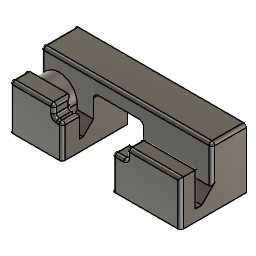
GBP - Cutting Tool v15 (Autodesk Fusion 360 design; units mm, degrees)
Autodesk Fusion 360 part; units mm, degrees
sketch "Boceto1" plane through (0, 0, 0) normal (0, 0, 1) x (1, 0, 0)
  line L0 (0, 7.25) -> (30, 7.25)
  line L1 (30, 7.25) -> (30, -4.25)
  line L2 (30, -4.25) -> (0, -4.25)
  line L3 (0, -4.25) -> (0, 7.25)
  dimension "d1" = 30
  dimension "d2" = 11.5
  dimension "d3" = 7.25
  constraint horizontal L0
  constraint vertical L1
  constraint horizontal L2
  constraint vertical L3
  measures "d1" distance of L0.start L0.end
  measures "d2" distance of L0.end L1.end
  measures "d3" distance of origin L0.start
extrude "Extruir1" add sketch "Boceto1" along normal blind 2
sketch "Boceto2" plane through (0, 0, 2) normal (0, 0, 1) x (-1, 0, 0)
  line L0 (0, 4.25) -> (-30, 4.25)
  line L1 (-30, 4.25) -> (-30, -7.25)
  line L2 (-30, -7.25) -> (0, -7.25)
  line L3 (0, -7.25) -> (0, 4.25)
  line L4 (0, -1.23) -> (-30, -1.23)
  line L5 (0, 1.23) -> (-30, 1.23)
  line L6 (-6.35, -1.23) -> (-6.35, 1.23)
  line L7 (-9.2, -1.23) -> (-9.2, 1.23)
  line L8 (-18, -1.23) -> (-18, 1.23)
  line L9 (0, -0.5) -> (-30, -0.5)
  dimension "d6" = 2.46
  dimension "d7" = 1.23
  dimension "d8" = 6.35
  dimension "d9" = 9.2
  dimension "d10" = 18
  constraint coincident L3 L4.start
  constraint coincident L1 L4.end
  constraint perpendicular L1 L4
  constraint coincident L3 L5.start
  constraint coincident L1 L5.end
  constraint perpendicular L1 L5
  constraint coincident L4 L6.start
  constraint coincident L5 L6.end
  constraint perpendicular L5 L6
  constraint coincident L4 L7.start
  constraint coincident L5 L7.end
  constraint perpendicular L5 L7
  constraint coincident L4 L8.start
  constraint coincident L5 L8.end
  constraint perpendicular L5 L8
  constraint coincident L3 L9.start
  constraint coincident L1 L9.end
  constraint perpendicular L1 L9
  measures "d6" distance of L4.end L5.end
  measures "d7" distance of origin L4.start
  measures "d8" horizontal distance of L2.end L6.start
  measures "d9" horizontal distance of L2.end L7.start
  measures "d10" horizontal distance of L2.end L8.start
extrude "Extruir2" add sketch "Boceto2" along normal blind 5.9 contours L3 L5 L6 L9 | L3 L4 L6 L9
sketch "Boceto3" plane through (0, -1.23, 0) normal (0, -1, 0) x (1, 0, 0)
  line L0 (0, 2) -> (6.35, 2)
  line L1 (6.35, 2) -> (6.35, 7.9)
  line L2 (6.35, 7.9) -> (0, 7.9)
  line L3 (0, 7.9) -> (0, 2)
  arc A0 (6.35, 4.725) -> (0, 4.725) centre (3.175, 4.725) ccw
  point P0 (3.175, 4.725)
  dimension "d13" = 3.175
  dimension "d14" = 3.175
  dimension "d54" = 3.175
  dimension "d55" = 3.175
  constraint coincident P0 A0.centre
  constraint coincident L3 A0.end
  constraint coincident L1 A0.start
  measures "d13" horizontal distance of L2.end P0
  measures "d14" vertical distance of L2.end P0
  measures "d54" distance of L2.end A0.end
  measures "d55" distance of L1.end A0.start
extrude "Extruir3" cut sketch "Boceto3" against normal blind 3 contours L2 L3 A0 | L1 L2 A0
extrude "Extruir4" cut sketch "Boceto2" against normal blind 2 contours L5 L7 L8 L9 | L4 L7 L8 L9
extrude "Extruir5" add sketch "Boceto2" along normal blind 5.9 contours L0 L1 L3 L5 | L1 L2 L3 L4
chamfer "Chaflán1" distance 1.8 angle 45 2 edges at (7.775, 1.23, 2) (24, 1.23, 2)
sketch "Boceto4" plane through (0, -1.23, 0) normal (0, 1, 0) x (-1, 0, 0)
  line L0 (-18, 2) -> (-18, 0)
  line L1 (-18, 0) -> (-9.2, 0)
  line L2 (-9.2, 0) -> (-9.2, 2)
  line L3 (-9.2, 2) -> (-6.35, 2)
  line L4 (-6.35, 2) -> (-6.35, 4.725)
  arc A0 (-3.175, 7.9) -> (-6.35, 4.725) centre (-3.175, 4.725) ccw
  line L5 (-3.175, 7.9) -> (-30, 7.9)
  line L6 (-30, 7.9) -> (-30, 2)
  line L7 (-30, 2) -> (-18, 2)
  line L8 (-9.2, 2) -> (-18, 2)
  constraint coincident L2.end L3.start
  constraint coincident L0.start L7.end
extrude "Extruir6" cut sketch "Boceto4" against normal blind 5 contours L0 L1 L2 L8
sketch "Boceto5" plane through (0, 1.23, 0) normal (0, -1, 0) x (1, 0, 0)
  line L0 (9.2, 3.8) -> (9.2, 0)
  line L1 (9.2, 0) -> (18, 0)
  line L2 (18, 0) -> (18, 3.8)
  line L3 (30, 3.8) -> (30, 7.9)
  line L4 (30, 7.9) -> (3.175, 7.9)
  arc A0 (6.35, 4.725) -> (3.175, 7.9) centre (3.175, 4.725) ccw
  line L5 (6.35, 4.725) -> (6.35, 3.8)
  line L6 (18, 3.8) -> (9.2, 3.8)
  line L7 (18, 3.8) -> (30, 3.8)
  line L8 (6.35, 3.8) -> (9.2, 3.8)
  constraint coincident L2.end L6.start
  constraint coincident L0.start L6.end
extrude "Extruir7" cut sketch "Boceto5" against normal blind 7 contours L0 L1 L2 L6
extrude "Extruir8" cut 2 faces at (15.0667, -2.2367, 2) (12.1333, 5.2433, 3.8) along direction (0, 0, 1) blind 4
extrude "Extruir10" add 1 faces at (11.0583, 5.2433, 7.9) along direction (0, 0, 1) blind 2.5
sketch "Boceto8" plane through (0, 0, 7.9) normal (0, 0, 1) x (-1, 0, 0)
  line L0 (-3.175, 1.23) -> (0, 1.23)
  line L1 (0, 1.23) -> (0, 4.25)
  line L2 (0, 4.25) -> (-30, 4.25)
  line L3 (-30, 4.25) -> (-30, 1.23)
  line L4 (-30, 1.23) -> (-3.175, 1.23)
  line L5 (-7.7, 1.23) -> (-7.7, 4.25)
  line L6 (-20.5, 1.23) -> (-20.5, 4.25)
  point P0 (0, 4.25)
  point P1 (-9.2, 4.25)
  point P2 (-18, 4.25)
  point P3 (-30, 4.25)
  dimension "d41" = 9.2
  dimension "d42" = 7.7
  dimension "d43" = 12
  dimension "d44" = 9.5
  constraint coincident L4 L5.start
  constraint coincident L2 L5.end
  constraint perpendicular L2 L5
  constraint coincident L4 L6.start
  constraint coincident L2 L6.end
  constraint perpendicular L2 L6
  measures "d41" distance of P0 P1
  measures "d42" distance of L5.end P0
  measures "d43" distance of P2 P3
  measures "d44" distance of L6.end P3
extrude "Extruir12" cut sketch "Boceto8" against normal blind 2 contours L2 L4 L5 L6
fillet "Empalme4" radius 0.5 29 edges at (0, -2.74, 7.9) (3.85, -4.25, 7.9) (7.7, -2.74, 7.9) (7.7, -4.25, 6.9) (7.7, -1.23, 6.9) (7.7, -2.74, 5.9) (8.45, -1.23, 5.9) (8.45, -4.25, 5.9) (9.2, -2.74, 5.9) (19.25, -1.23, 5.9) (18, -2.74, 5.9) (19.25, -4.25, 5.9) (20.5, -2.74, 7.9) (25.25, -1.23, 7.9) (25.25, -4.25, 7.9) (20.5, -1.23, 6.9) (20.5, -4.25, 6.9) (20.5, -2.74, 5.9) (15, 1.23, 10.4) (0, 4.24, 10.4) (30, 4.24, 10.4) (0, -4.25, 3.95) (9.2, -4.25, 2.95) (18, -4.25, 2.95) (30, -4.25, 3.95) (0, 1.23, 7.5625) (30, 1.23, 7.1) (30, -1.23, 4.95) (0, -1.23, 6.3125)
fillet "Empalme5" radius 0.8 2 edges at (9.2, 4.24, 7.8) (18, 4.24, 7.8)
equation "d3 = d2 / 2 + 1.5 mm"
equation "d7 = d6 / 2"
equation "d9 = d10 - 8.8 mm"
equation "d13 = d8 / 2"
equation "d14 = d13"
equation "d42 = d41 - 1.5 mm"
equation "d44 = d43 - 2.5 mm"
equation "d54 = d8 / 2"
equation "d55 = d8 / 2"
